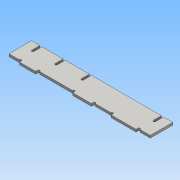
# Autodesk Inventor part: Board_separator
Saved by Autodesk Inventor 2016 (Build 200138000, 138)
## iProperties
Created: 2016-03-29
Part Number: Board_separator
Material: Generic
Document SubType Name: Modeling
Designer: admin
Density: 1 g/cm^3
Appearance: Default
Author: admin
Autodesk Inventor part; units mm, degrees
ref_plane "YZ Plane" through (0, 0, 0) normal (1, 0, 0) x (0, 1, 0)
ref_plane "XZ Plane" through (0, 0, 0) normal (0, 1, 0) x (-1, 0, 0)
ref_plane "XY Plane" through (0, 0, 0) normal (0, 0, 1) x (1, 0, 0)
sketch "Sketch4" plane through (0, 0, 0) normal (0, 0, 1) x (1, 0, 0)
  line L0 (-60.5, 9.1) -> (-60.5, -9.1)
  line L1 (53.5, 9.1) -> (53.5, -9.1)
  line L2 (-37.5, -10.6) -> (-37.5, -9.1)
  line L3 (-50.5, -9.1) -> (-50.5, -10.6)
  line L4 (-52.3, -9.1) -> (-60.5, -9.1)
  line L5 (-35.7, -9.1) -> (-9.3, -9.1)
  line L6 (-7.5, -9.1) -> (-7.5, -10.6)
  line L7 (23.5, -10.6) -> (23.5, -9.1)
  line L8 (43.5, -9.1) -> (43.5, -10.6)
  line L9 (45.3, -9.1) -> (53.5, -9.1)
  line L10 (21.7, -9.1) -> (9.3, -9.1)
  line L11 (7.5, -9.1) -> (7.5, -10.6)
  line L12 (-50.5, -10.6) -> (-37.5, -10.6)
  line L13 (-7.5, -10.6) -> (7.5, -10.6)
  line L14 (23.5, -10.6) -> (43.5, -10.6)
  arc A0 (-50.5, -9.1) -> (-52.3, -9.1) centre (-51.4, -9.1) ccw
  arc A1 (-35.7, -9.1) -> (-37.5, -9.1) centre (-36.6, -9.1) ccw
  arc A2 (-7.5, -9.1) -> (-9.3, -9.1) centre (-8.4, -9.1) ccw
  arc A3 (9.3, -9.1) -> (7.5, -9.1) centre (8.4, -9.1) ccw
  arc A4 (23.5, -9.1) -> (21.7, -9.1) centre (22.6, -9.1) ccw
  arc A5 (45.3, -9.1) -> (43.5, -9.1) centre (44.4, -9.1) ccw
  line L15 (-53.75, 9.1) -> (-53.75, 2.6)
  line L16 (-52.05, 2.6) -> (-52.05, 9.1)
  line L17 (-35, 9.1) -> (-35, 2.6)
  line L18 (-33.3, 2.6) -> (-33.3, 9.1)
  line L19 (-13.8, 9.1) -> (-13.8, 2.6)
  line L20 (-12.1, 2.6) -> (-12.1, 9.1)
  line L21 (46.05, 9.1) -> (46.05, 2.6)
  line L22 (44.35, 2.6) -> (44.35, 9.1)
  line L23 (-53.75, 9.1) -> (-60.5, 9.1)
  line L24 (-35, 9.1) -> (-52.05, 9.1)
  line L25 (-13.8, 9.1) -> (-33.3, 9.1)
  line L26 (53.5, 9.1) -> (46.05, 9.1)
  line L27 (44.35, 9.1) -> (-12.1, 9.1)
  arc A6 (-53.75, 2.6) -> (-52.05, 2.6) centre (-52.9, 2.6) ccw
  arc A7 (-35, 2.6) -> (-33.3, 2.6) centre (-34.15, 2.6) ccw
  arc A8 (-13.8, 2.6) -> (-12.1, 2.6) centre (-12.95, 2.6) ccw
  arc A9 (44.35, 2.6) -> (46.05, 2.6) centre (45.2, 2.6) ccw
  point P0 (0, 0)
  point P1 (0, 9.1)
  point P2 (-60.5, 0)
  point P3 (0, -10.6)
  dimension "d25" = 10
  dimension "d26" = 13
  dimension "d27" = 30
  dimension "d28" = 10
  dimension "d29" = 114
  dimension "d33" = 1.5
  dimension "d36" = 1.8
  dimension "d37" = 20
  dimension "d38" = 15
  dimension "d39" = 16
  dimension "d41" = 1.7
  dimension "d44" = 19.5
  dimension "d45" = 17.05
  dimension "d46" = 56.45
  dimension "d48" = 6.75
  dimension "d49" = 18.2
  dimension "d51" = 6.5
  dimension "d52" = 1.7
  dimension "d53" = 1.7
  dimension "d54" = 1.7
  constraints: 56 end point, 21 perpendicular, 20 point on circle, 10 centre point, 10 tangent, 9 collinear, 8 horizontal alignment, 7 horizontal, 7 point on line, 5 equal radius, 5 vertical, 2 midpoint, 2 parallel, 2 vertical alignment
  measures "d25" distance between parallel lines of L3 L0
  measures "d26" distance between parallel lines of L2 L3
  measures "d27" distance of L2.end L6.start
  measures "d28" distance between parallel lines of L1 L8
  measures "d29" distance of L1.start L0.start
  measures "d33" distance between parallel lines of L12 L4
  measures "d36" diameter of A0
  measures "d37" distance between parallel lines of L8 L7
  measures "d38" distance between parallel lines of L11 L6
  measures "d39" distance between parallel lines of L7 L11
  measures "d41" distance between parallel lines of L16 L15
  measures "d44" distance between parallel lines of L19 L18
  measures "d45" distance between parallel lines of L17 L16
  measures "d46" distance between parallel lines of L22 L20
  measures "d48" distance of L15.start L0.start
  measures "d49" distance between parallel lines of L4 L23
  measures "d51" distance from line of L23 A6.centre
  measures "d52" distance between parallel lines of L18 L17
  measures "d53" distance between parallel lines of L20 L19
  measures "d54" distance between parallel lines of L21 L22
extrude "Extrusion2" add sketch "Sketch4" along normal blind 2
equation "\"d52\" = d41"
equation "\"d53\" = d52"
equation "\"d54\" = d53"
body "Solid1"
